esp32_ttgo (Autodesk Fusion 360 design; units mm, degrees)
Autodesk Fusion 360 part; units mm, degrees
sketch "Sketch1" plane through (0, 0, 0) normal (1, 0, 0) x (0, 1, 0)
  line L0 (0, 0) -> (-51.5, 0)
  line L1 (-51.5, 0) -> (-51.5, 25.3)
  line L2 (-51.5, 25.3) -> (0, 25.3)
  line L3 (0, 25.3) -> (0, 0)
  dimension "d1" = 25.3
  dimension "d2" = 51.5
  constraint horizontal L0
  constraint vertical L1
  constraint horizontal L2
  constraint vertical L3
  constraint coincident L0.start L3.end
  measures "d1" distance of L0.start L2.end
  measures "d2" distance of L1.end L2.end
extrude "Extrude1" add sketch "Sketch1" along normal blind 1.2 makes body 1
sketch "Sketch2" plane through (0, -51.5, 0) normal (0, -1, 0) x (1, 0, 0)
  line L0 (0, 25.3) -> (0, 0)
  line L1 (0, 0) -> (1.2, 0)
  line L2 (1.2, 0) -> (1.2, 25.3)
  line L3 (1.2, 25.3) -> (0, 25.3)
  line L4 (1.2, 17.15) -> (4.5, 17.15)
  line L5 (4.5, 17.15) -> (4.5, 8.15)
  line L6 (4.5, 8.15) -> (1.2, 8.15)
  line L7 (1.2, 8.15) -> (1.2, 17.15)
  line L8 (4.5, 12.65) -> (1.2, 12.65)
  line L9 (1.2, 25.3) -> (1.2, 0)
  dimension "d5" = 9
  dimension "d7" = 4.5
  constraint horizontal L4
  constraint vertical L5
  constraint horizontal L6
  constraint vertical L7
  constraint coincident L2 L4.start
  constraint midpoint L5 L8.start
  constraint midpoint L7 L8.end
  constraint coincident L2.end L3.start
  constraint coincident L1.end L2.start
  constraint midpoint L8.end L9
  measures "d5" distance of L4.end L5.end
  measures "d7" distance of L0 L5
extrude "Extrude2" add sketch "Sketch2" along normal blind 1.1 and the other way blind 6 separate body contours L2 L4 L5 L7 L8 L9 | L2 L5 L6 L7 L8 L9 makes body 2
sketch "Sketch3" plane through (1.2, 0, 0) normal (1, 0, 0) x (0, 1, 0)
  line L0 (0, 25.3) -> (-51.5, 25.3)
  line L1 (-51.5, 25.3) -> (-51.5, 0)
  line L2 (-51.5, 0) -> (0, 0)
  line L3 (0, 0) -> (0, 25.3)
  line L4 (-50.5, 22.9) -> (-46.3, 22.9)
  line L5 (-46.3, 22.9) -> (-46.3, 19.5)
  line L6 (-46.3, 19.5) -> (-50.5, 19.5)
  line L7 (-50.5, 19.5) -> (-50.5, 22.9)
  line L8 (0, 12.65) -> (-51.5, 12.65)
  line L9 (-46.3, 2.4) -> (-46.3, 5.8)
  line L10 (-50.5, 2.4) -> (-46.3, 2.4)
  line L11 (-50.5, 5.8) -> (-50.5, 2.4)
  line L12 (-46.3, 5.8) -> (-50.5, 5.8)
  dimension "d12" = 3.4
  dimension "d13" = 4.2
  dimension "d14" = 2.4
  dimension "d15" = 1
  constraint horizontal L4
  constraint vertical L5
  constraint horizontal L6
  constraint vertical L7
  constraint midpoint L3 L8.start
  constraint midpoint L1 L8.end
  constraint symmetric L4.start L8 L10.start
  constraint symmetric L4.end L8 L9.start
  constraint symmetric L5.end L8 L9.end
  constraint symmetric L6.end L8 L11.start
  measures "d12" distance of L4.end L5.end
  measures "d13" distance of L4.start L4.end
  measures "d14" distance of L0 L4
  measures "d15" distance of L1 L7
extrude "Extrude3" add sketch "Sketch3" along normal blind 2.6 contours L4 L5 L6 L7 | L9 L10 L11 L12 bodies 1
sketch "Sketch4" plane through (0, 0, 0) normal (-1, 0, 0) x (0, -1, 0)
  line L0 (51.5, 25.3) -> (0, 25.3)
  line L1 (0, 25.3) -> (0, 0)
  line L2 (0, 0) -> (51.5, 0)
  line L3 (51.5, 0) -> (51.5, 25.3)
  line L4 (40.9, 16.45) -> (45.5, 16.45)
  line L5 (45.5, 16.45) -> (45.5, 8.85)
  line L6 (45.5, 8.85) -> (40.9, 8.85)
  line L7 (40.9, 8.85) -> (40.9, 16.45)
  line L8 (51.5, 25.3) -> (51.5, 0)
  line L9 (40.9, 12.65) -> (45.5, 12.65)
  line L10 (51.5, 12.65) -> (0, 12.65)
  dimension "d18" = 7.6
  dimension "d19" = 4.6
  dimension "d20" = 6
  constraint horizontal L4
  constraint vertical L5
  constraint horizontal L6
  constraint vertical L7
  constraint coincident L0.start L3.end
  constraint coincident L2.end L3.start
  constraint midpoint L7 L9.start
  constraint midpoint L5 L9.end
  constraint midpoint L8 L10.start
  constraint collinear L9 L10
  constraint midpoint L1 L10.end
  measures "d18" distance of L4.end L5.end
  measures "d19" distance of L4.start L4.end
  measures "d20" distance of L5 L8
extrude "Extrude4" add sketch "Sketch4" along normal blind 3.4 contours L4 L5 L7 L9 L10 | L5 L6 L7 L9 L10 bodies 1
sketch "Sketch5" plane through (1.2, 0, 0) normal (1, 0, 0) x (0, 1, 0)
  line L0 (-46.3, 5.8) -> (-46.3, 2.4)
  line L1 (-46.3, 2.4) -> (-50.5, 2.4)
  line L2 (-50.5, 2.4) -> (-50.5, 5.8)
  line L3 (-50.5, 5.8) -> (-46.3, 5.8)
  line L4 (-50.5, 19.5) -> (-50.5, 22.9)
  line L5 (-50.5, 22.9) -> (-46.3, 22.9)
  line L6 (-46.3, 22.9) -> (-46.3, 19.5)
  line L7 (-46.3, 19.5) -> (-50.5, 19.5)
  line L8 (0, 25.3) -> (-51.5, 25.3)
  line L9 (-51.5, 25.3) -> (-51.5, 0)
  line L10 (-51.5, 0) -> (0, 0)
  line L11 (0, 0) -> (0, 25.3)
  line L12 (-41.9, 0) -> (-37.3, 0)
  line L13 (-37.3, 0) -> (-37.3, 2.3)
  line L14 (-37.3, 2.3) -> (-41.9, 2.3)
  line L15 (-41.9, 2.3) -> (-41.9, 0)
  dimension "d23" = 4.6
  dimension "d24" = 2.3
  dimension "d25" = 14.2
  constraint horizontal L12
  constraint vertical L13
  constraint horizontal L14
  constraint vertical L15
  constraint coincident L10 L12.start
  measures "d23" distance of L13.end L14.end
  measures "d24" distance of L12.start L14.end
  measures "d25" distance of L9 L13
extrude "Extrude5" add sketch "Sketch5" along normal blind 1.9 contours L10 L12 L13 L14 L15 bodies 1
sketch "Sketch6" plane through (0, 0, 0) normal (0, 0, -1) x (1, 0, 0)
  line L0 (0, 51.5) -> (0, 0)
  line L1 (0, 0) -> (1.2, 0)
  line L2 (1.2, 0) -> (1.2, 37.3)
  line L3 (1.2, 37.3) -> (3.1, 37.3)
  line L4 (3.1, 37.3) -> (3.1, 41.9)
  line L5 (3.1, 41.9) -> (1.2, 41.9)
  line L6 (1.2, 41.9) -> (1.2, 51.5)
  line L7 (1.2, 51.5) -> (0, 51.5)
  line L8 (1.6, 40.7) -> (2.6, 40.7)
  line L9 (2.6, 40.7) -> (2.6, 38.5)
  line L10 (2.6, 38.5) -> (1.6, 38.5)
  line L11 (1.6, 38.5) -> (1.6, 40.7)
  dimension "d28" = 1.2
  dimension "d29" = 1.2
  dimension "d30" = 0.5
  dimension "d31" = 1
  constraint horizontal L8
  constraint vertical L9
  constraint horizontal L10
  constraint vertical L11
  measures "d28" distance of L5 L8
  measures "d29" distance of L3 L10
  measures "d30" distance of L4 L9
  measures "d31" distance of L8.start L8.end
extrude "Extrude6" add sketch "Sketch6" along normal blind 1 contours L8 L9 L10 L11 bodies 1
sketch "Sketch7" plane through (0, 0, 0) normal (-1, 0, 0) x (0, -1, 0)
  line L0 (40.9, 8.85) -> (40.9, 16.45)
  line L1 (40.9, 16.45) -> (45.5, 16.45)
  line L2 (45.5, 16.45) -> (45.5, 8.85)
  line L3 (45.5, 8.85) -> (40.9, 8.85)
  line L4 (51.5, 25.3) -> (0, 25.3)
  line L5 (0, 25.3) -> (0, 0)
  line L6 (0, 0) -> (51.5, 0)
  line L7 (51.5, 0) -> (51.5, 25.3)
  line L8 (39.9, 25.3) -> (19.9, 25.3)
  line L9 (19.9, 25.3) -> (19.9, 2.2)
  line L10 (19.9, 2.2) -> (39.9, 2.2)
  line L11 (39.9, 2.2) -> (39.9, 25.3)
  line L12 (39.9, 25.3) -> (51.5, 25.3)
  line L13 (51.5, 25.3) -> (51.5, 0)
  line L14 (51.5, 0) -> (39.9, 0)
  line L15 (39.9, 0) -> (39.9, 25.3)
  line L16 (5.7, 23.1) -> (19.9, 23.1)
  line L17 (19.9, 23.1) -> (19.9, 2.2)
  line L18 (19.9, 2.2) -> (5.7, 2.2)
  line L19 (5.7, 2.2) -> (5.7, 23.1)
  line L20 (19.9, 23.1) -> (36, 23.1)
  line L21 (36, 23.1) -> (36, 25.3)
  dimension "d34" = 1
  dimension "d35" = 20
  dimension "d36" = 2.2
  dimension "d37" = 5.7
  dimension "d38" = 2.2
  dimension "d39" = 2.2
  dimension "d40" = 36
  constraint horizontal L8
  constraint vertical L9
  constraint horizontal L10
  constraint vertical L11
  constraint horizontal L12
  constraint vertical L13
  constraint horizontal L14
  constraint vertical L15
  constraint horizontal L16
  constraint vertical L17
  constraint horizontal L18
  constraint vertical L19
  constraint collinear L7 L13
  constraint collinear L4 L12
  constraint collinear L6 L14
  constraint collinear L11 L15
  constraint collinear L4 L8
  constraint collinear L9 L17
  constraint perpendicular L9 L20
  constraint perpendicular L8 L21
  constraint coincident L8 L21.end
  measures "d34" distance of L0 L11
  measures "d35" distance of L9.end L10.end
  measures "d36" distance of L6 L10
  measures "d37" distance of L5 L19
  measures "d38" distance of L6 L18
  measures "d39" distance of L4 L16
  measures "d40" distance of L5 L21
extrude "Extrude7" add sketch "Sketch7" along normal blind 1.95 contours L4 L8 L9 L10 L11 L15 L17 L20 L21 bodies 1
extrude "Extrude8" add sketch "Sketch7" along normal blind 0.9 contours L4 L6 L7 L11 L12 L13 L14 L15 | L9 L16 L17 L18 L19 bodies 1
sketch "Sketch8" plane through (1.2, 0, 0) normal (1, 0, 0) x (0, 1, 0)
  line L0 (-37.3, 2.3) -> (-37.3, 0)
  line L1 (-37.3, 0) -> (0, 0)
  line L2 (0, 0) -> (0, 25.3)
  line L3 (0, 25.3) -> (-51.5, 25.3)
  line L4 (-51.5, 25.3) -> (-51.5, 0)
  line L5 (-51.5, 0) -> (-41.9, 0)
  line L6 (-41.9, 0) -> (-41.9, 2.3)
  line L7 (-41.9, 2.3) -> (-37.3, 2.3)
  line L8 (-46.3, 5.8) -> (-46.3, 2.4)
  line L9 (-46.3, 2.4) -> (-50.5, 2.4)
  line L10 (-50.5, 2.4) -> (-50.5, 5.8)
  line L11 (-50.5, 5.8) -> (-46.3, 5.8)
  line L12 (-50.5, 19.5) -> (-50.5, 22.9)
  line L13 (-50.5, 22.9) -> (-46.3, 22.9)
  line L14 (-46.3, 22.9) -> (-46.3, 19.5)
  line L15 (-46.3, 19.5) -> (-50.5, 19.5)
  line L16 (-51.5, 25.3) -> (-39, 25.3)
  line L17 (-39, 25.3) -> (-39, 0)
  line L18 (-39, 0) -> (-51.5, 0)
  line L19 (-51.5, 0) -> (-51.5, 25.3)
  dimension "d45" = 12.5
  constraint horizontal L16
  constraint vertical L17
  constraint horizontal L18
  constraint vertical L19
  constraint coincident L3.end L4.start
  measures "d45" distance of L3.end L16.end
extrude "Extrude9" add sketch "Sketch8" along normal blind 1 contours L3 L4 L5 L6 L7 L16 L17 L18 L19 bodies 2 1
equation "d38 = d36"
equation "d39 = d38"
equation "d41 = 3.15 mm - 1.2 mm"
equation "d43 = 2.1 mm - 1.2 mm"
